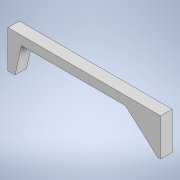
# Autodesk Inventor part: vydacha_6
Saved by Autodesk Inventor 2020 (Build 240168000, 168)
## iProperties
Created: 2022-07-27
Part Number: vydacha_6
Material: Типовые
Document SubType Name: Modeling
Designer: akapu
Density: 1 g/cm^3
Appearance: По умолчанию
Author: akapu
Autodesk Inventor part; units mm, degrees
ref_plane "YZ Plane" through (0, 0, 0) normal (1, 0, 0) x (0, 1, 0)
ref_plane "XZ Plane" through (0, 0, 0) normal (0, 1, 0) x (-1, 0, 0)
ref_plane "XY Plane" through (0, 0, 0) normal (0, 0, 1) x (1, 0, 0)
sketch "Эскиз1" plane through (0, 0, 0) normal (0, 0, 1) x (1, 0, 0)
  line L0 (0, 0) -> (0, 6.146)
  line L1 (0, 0) -> (72.5, 0)
  line L2 (72.5, 0) -> (72.5, 6.146)
  line L3 (72.5, 6.146) -> (0, 6.146)
  line L4 (95, -20) -> (72.5, 0)
  line L5 (-4.5, -20) -> (0, 0)
  line L6 (-4.5, -20) -> (-9.5, -20)
  line L7 (-9.5, -20) -> (-9.5, 6.146)
  line L8 (-9.5, 6.146) -> (0, 6.146)
  line L9 (95, -20) -> (97, -20)
  line L10 (97, -20) -> (97, 6.146)
  line L11 (97, 6.146) -> (72.5, 6.146)
  point P0 (100, 6.146)
  dimension "d0" = 6.146
  dimension "d1" = 72.5
  dimension "d5" = 5
  dimension "d9" = 2
  constraints: 24 end point, 4 perpendicular, 3 horizontal, 1 point on line, 1 vertical
  measures "d0" distance of L0.start L0.end
  measures "d1" distance of L0.start L1.end
  measures "d5" distance of L5.start L6.end
  measures "d9" distance of L4.start L9.end
extrude "Выдавливание1" add sketch "Эскиз1" along normal blind 8
